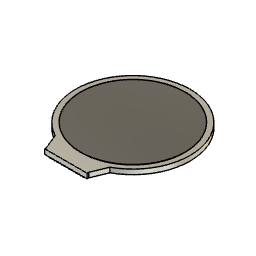
FocKnob v35 (Autodesk Fusion 360 archive; units mm, degrees)
design "TFT-Round-1.28"
Autodesk Fusion 360 part; units mm, degrees
sketch "Sketch1" plane through (0, 0, 0) normal (0, 0, 1) x (1, 0, 0)
  circle A0 centre (0, 0) radius 16.2
  circle A1 centre (0, 0) radius 17.37 construction
  circle A2 centre (0, 0) radius 17.6 construction
  circle A3 centre (0, 0) radius 17.8
  line L0 (0, 0) -> (0, -34.4204) construction
  line L1 (-6.6, -20.3) -> (6.6, -20.3)
  line L2 (8.5, -15.6394) -> (-8.5, -15.6394) construction
  line L3 (6.6, -20.3) -> (8.5, -15.6394)
  line L4 (-6.6, -20.3) -> (-8.5, -15.6394)
  line L5 (-6.6, -20.3) -> (-6.6, -20.8)
  line L6 (-6.6, -20.8) -> (6.6, -20.8)
  line L7 (6.6, -20.8) -> (6.6, -20.3)
  circle A4 centre (0, 0) radius 22.5 construction
  line L8 (-5.7, -20.8) -> (5.7, -20.8)
  line L9 (5.7, -20.8) -> (5.7, -10.06)
  line L10 (5.7, -10.06) -> (-5.7, -10.06)
  line L11 (-5.7, -10.06) -> (-5.7, -20.8)
  point P0 (0, -20.3)
  dimension "d1" = 32.4
  dimension "d2" = 34.74
  dimension "d3" = 35.2
  dimension "d4" = 35.6
  dimension "d5" = 13.2
  dimension "d6" = 20.3
  dimension "d7" = 17
  dimension "d8" = 0.5
  dimension "d9" = 21.822
  dimension "d10" = 45
  dimension "d11" = 0.678
  dimension "d24" = 11.4
  dimension "d25" = 10.24
  constraint coincident A0.centre A1.centre
  constraint concentric A0 A1
  constraint concentric A1 A2
  constraint concentric A0 A3
  constraint vertical L0
  constraint horizontal L1
  constraint midpoint L1 P0
  constraint coincident L0 P0
  constraint coincident A3 L2.start
  constraint coincident A3 L2.end
  constraint horizontal L2
  constraint perpendicular L1 L5
  constraint perpendicular L5 L6
  constraint vertical L7
  constraint concentric A0 A4
  constraint horizontal L8
  constraint vertical L9
  constraint horizontal L10
  constraint vertical L11
  constraint coincident L6 L8.start
  constraint midpoint L6 L8
  measures "d1" diameter of A0
  measures "d2" diameter of A1
  measures "d3" diameter of A2
  measures "d4" diameter of A3
  measures "d5" distance of L1.start L1.end
  measures "d6" distance of A0.centre L1
  measures "d7" distance of L2.start L2.end
  measures "d8" distance of L1 L6
  measures "d9" distance of A0.centre L6.end
  measures "d10" diameter of A4
  measures "d11" distance of L6.end A4
  measures "d24" distance of L8.start L8.end
  measures "d25" distance of L1 L10
extrude "Extrude2" add sketch "Sketch1" along normal blind 1.5 makes body 1
extrude "Extrude4" add sketch "Sketch1" along normal blind 0.1 from surface at 1.5 contours A0 L9 L10 L11 | A0 L9 L10 L11 bodies 1
extrude "Extrude5" add sketch "Sketch1" against normal blind 0.13 separate body contours A0 L9 L10 L11 | A0 A3 L9 L11 | A3 L1 L9 L11 | L1 L6 L8 L9 L11 picked at (0.388, -12.0927) picked at (-4.9559, -15.9504) makes body 2
equation "d6 = 38.1 mm - d4 / 2"
named bodies: "LCd", "FPC"
